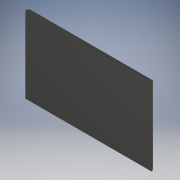
# Autodesk Inventor part: BA03
Saved by Autodesk Inventor 2017 (Build 210142000, 142)
## iProperties
Created: 2018-10-18
Part Number: BA03
Material: ABS Plastic
Document SubType Name: Modeling
Designer: Dell
Density: 1.06 g/cm^3
Appearance: Smooth - Black
Author: Dell
Autodesk Inventor part; units mm, degrees
ref_plane "YZ Plane" through (0, 0, 0) normal (1, 0, 0) x (0, 1, 0)
ref_plane "XZ Plane" through (0, 0, 0) normal (0, 1, 0) x (-1, 0, 0)
ref_plane "XY Plane" through (0, 0, 0) normal (0, 0, 1) x (1, 0, 0)
sketch "Sketch1" plane through (0, 0, 0) normal (0, 0, 1) x (1, 0, 0)
  line L0 (0, 0) -> (303.5592, 0)
  line L1 (303.5592, 0) -> (303.5592, -184.15)
  line L2 (303.5592, -184.15) -> (0, -184.15)
  line L3 (0, -184.15) -> (0, 0)
  line L4 (455.3388, 262.89) -> (303.5592, 0)
  line L5 (303.5592, 0) -> (0, 0)
  line L6 (0, 0) -> (-151.7796, 262.89)
  line L7 (-151.7796, 262.89) -> (0, 525.78)
  line L8 (0, 525.78) -> (303.5592, 525.78)
  line L9 (303.5592, 525.78) -> (455.3388, 262.89)
  point P0 (151.7796, 262.89)
  dimension "d1" = 184.15
  dimension "d18" = 525.78
  constraints: 20 end point, 2 parallel, 1 horizontal, 1 perpendicular, 13 other
  measures "d1" distance of L0.end L1.end
  measures "d18" distance between parallel lines of L4 L7
extrude "Extrusion1" add sketch "Sketch1" along normal blind 6.35 contours L0 L1 L2 L3
sketch "Sketch4" plane through (0, 0, 0) normal (0, 1, 0) x (1, 0, 0)
  line L0 (303.5592, -6.35) -> (0, -6.35) construction
  line L1 (0, -6.35) -> (3.6662, 0)
  line L2 (0, 0) -> (303.5592, 0) construction
  line L3 (0, 0) -> (3.6662, 0)
  line L4 (0, 0) -> (0, -6.35) projected
  line L5 (0, -6.35) -> (0, 0)
  line L6 (303.5592, 0) -> (303.5592, -6.35) projected
  line L7 (303.5592, -6.35) -> (299.8931, 0)
  line L8 (299.8931, 0) -> (303.5592, 0)
  line L9 (303.5592, 0) -> (303.5592, -6.35)
  dimension "d19" = 30
  dimension "d20" = 30
  constraints: 12 end point, 2 collinear, 2 point on line
  measures "d19" angle of L6 L7
  measures "d20" angle of L4 L1
extrude "Extrusion4" cut sketch "Sketch4" against normal through all
sketch "Sketch5" plane through (0, 0, 6.35) normal (0, 0, 1) x (1, 0, 0)
  line L0 (3.6662, 0) -> (299.8931, 0) projected
  line L1 (151.7796, 0) -> (151.7796, -72.075)
  line L2 (151.7796, -72.075) -> (131.7796, -92.075)
  line L3 (131.7796, -92.075) -> (151.7796, -112.075)
  line L4 (151.7796, -112.075) -> (151.7796, -184.15)
  line L5 (0, -184.15) -> (303.5592, -184.15) projected
  line L6 (151.7796, -184.15) -> (0, -184.15)
  line L7 (0, -184.15) -> (0, 0)
  line L8 (3.6662, -184.15) -> (3.6662, 0) projected
  line L9 (0, 0) -> (151.7796, 0)
  line L10 (151.7796, 0) -> (303.5592, 0)
  line L11 (303.5592, 0) -> (303.5592, -184.15)
  line L12 (303.5592, -184.15) -> (151.7796, -184.15)
  line L13 (151.7796, -184.15) -> (151.7796, 0)
  point P0 (0, -92.075)
  dimension "d23" = 40
  dimension "d24" = 20
  constraints: 22 end point, 3 midpoint, 3 parallel, 2 collinear, 2 perpendicular, 2 point on line, 1 horizontal, 1 horizontal alignment, 1 vertical
  measures "d23" distance of L1.end L3.end
  measures "d24" distance from line of L1 L2.end
extrude "Extrusion5" [suppressed]
body "Solid1"
